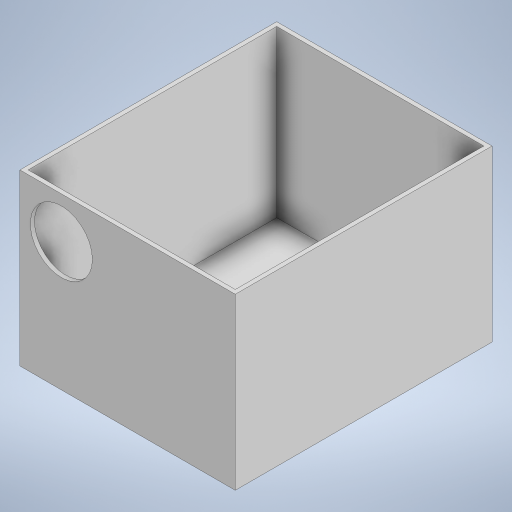
# Autodesk Inventor part: Part4 zaid
Saved by Autodesk Inventor 2023 (Build 270158030, 158C)
## iProperties
Created: 2023-04-28
Part Number: Part4 zaid
Material: Generic
Document SubType Name: Modeling
Designer: 22165
Density: 1 g/cm^3
Appearance: Default
Author: 22165
Autodesk Inventor part; units mm, degrees
ref_plane "YZ Plane" through (0, 0, 0) normal (1, 0, 0) x (0, 1, 0)
ref_plane "XZ Plane" through (0, 0, 0) normal (0, 1, 0) x (-1, 0, 0)
ref_plane "XY Plane" through (0, 0, 0) normal (0, 0, 1) x (1, 0, 0)
sketch "Sketch1" plane through (0, 0, 0) normal (0, 0, 1) x (1, 0, 0)
  line L0 (0, 0) -> (50, 0)
  line L1 (50, 0) -> (50, -40)
  line L2 (50, -40) -> (0, -40)
  line L3 (0, -40) -> (0, 0)
  dimension "d0" = 50
  dimension "d1" = 40
  constraints: 8 end point, 2 parallel, 1 horizontal, 1 perpendicular
  measures "d0" distance of L1.end L2.end
  measures "d1" distance of L0.end L1.end
extrude "Extrusion1" add sketch "Sketch1" along normal blind 60
shell "Shell1" thickness 1 outward yes removed faces 1 at (33.3333, 0, 20)
sketch "Sketch2" plane through (0, 0, 61) normal (0, 0, 1) x (1, 0, 0)
  circle A0 centre (9, -10) radius 7.5
  line L0 (51, 0) -> (-1, 0) projected
  line L1 (-1, 0) -> (-1, -41) projected
  point P0 (0, 0)
  dimension "d5" = 10
  dimension "d6" = 10
  dimension "d7" = 15
  constraints: 1 centre point
  measures "d5" distance from line of L0 A0.centre
  measures "d6" distance from line of L1 A0.centre
  measures "d7" diameter of A0
extrude "Extrusion2" cut sketch "Sketch2" against normal blind 60
body "Solid1"
